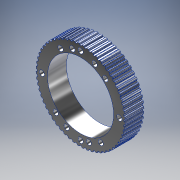
# Autodesk Inventor part: Synchronous Pulley1
Saved by Autodesk Inventor 2019.4 (Build 234330000, 330)
## iProperties
Created: 2019-11-30
Part Number: Synchronous Pulley1
Material: Aluminum 6061
Document SubType Name: Modeling
Designer: admin
Density: 2.7 g/cm^3
Appearance: Aluminum - Flat
Mass: 156.055 g
Surface Area: 190.164 cm^2
Volume: 57.7982 cm^3
CustomPartVersion: 1
Author: admin
Autodesk Inventor part; units mm, degrees
ref_plane "YZ Plane" through (0, 0, 0) normal (1, 0, 0) x (0, 1, 0)
ref_plane "XZ Plane" through (0, 0, 0) normal (0, 1, 0) x (-1, 0, 0)
ref_plane "XY Plane" through (0, 0, 0) normal (0, 0, 1) x (1, 0, 0)
sketch "Pulley Sketch" plane through (0, 0, 0) normal (0, 0, 1) x (1, 0, 0)
  circle A0 centre (0, 0) radius 47.7465 construction
  circle A1 centre (0, 0) radius 47.2465
  circle A2 centre (0, 0) radius 45.9965
  line L0 (-1.4722, 47.2235) -> (-0.9, 45.9965)
  line L1 (-0.9, 45.9965) -> (0.9, 45.9965)
  line L2 (0.9, 45.9965) -> (1.4722, 47.2235)
  line L3 (0, 0) -> (0, 47.2465) construction
  point P0 (0, 45.9965)
  dimension "d0" = 95.493
  dimension "d1" = 0.5
  dimension "d2" = 1.25
  dimension "d3" = 50
  dimension "d4" = 1.8
  constraints: 8 end point, 3 coincident, 3 point on circle, 2 centre point, 1 horizontal, 1 midpoint, 1 point on line, 1 vertical, 1 vertical alignment, 3 other
  measures "d0" diameter of A0
  measures "d1" radial gap between concentric circles of A0 A1
  measures "d3" angle of L2 L0
  measures "d4" distance of L0.end L1.end
extrude "Base Body" add sketch "Pulley Sketch" along normal mid plane 20 contours A2 | A1 L0 L1 L2 | L2 L1 L0 A1
extrude "Tooth" cut sketch "Pulley Sketch" along normal through all both and the other way through all contours L2 L1 L0 A1 picked at (0, 46.8281)
fillet "Tooth Fillet" radius 0.4 2 edges at (0.9, 45.9965, 0) (-0.9, 45.9965, 0)
fillet "Tooth Fillet" radius 0.6 4 edges at (-1.4722, 47.2235, 5) (-1.4722, 47.2235, -5) (1.4722, 47.2235, 5) (1.4722, 47.2235, -5)
pattern_circular "Teeth" count 60 over 360 about axis through (0, 0, -10) along (0, 0, 1) of "Tooth", "Tooth Fillet"
feature "Left flange" [suppressed]
feature "Right flange" [suppressed]
sketch "Sketch2" plane through (0, 0, 10) normal (0, 0, 1) x (1, 0, 0)
  arc A0 (-41.8204, 21.9837) -> (-42.3666, 20.9118) centre (0, 0) ccw projected
  constraints: 1 coincident
hole "Hole1" at (0, 0, 10) direction (0, 0, -1) diameter 70 end through all
sketch "Sketch3" plane through (0, 0, 10) normal (0, 0, 1) x (1, 0, 0)
  circle A0 centre (0, 41) radius 2.75
  line L0 (0, 41) -> (0, 0) construction
  circle A1 centre (-41, 0) radius 2.75
  circle A2 centre (0, -41) radius 2.75
  circle A3 centre (41, 0) radius 2.75
  dimension "d24" = 5.5
  dimension "d25" = 41
  dimension "d28" = 360
  constraints: 4 centre point, 2 end point, 1 vertical, 9 other
  measures "d24" diameter of A0
  measures "d25" distance of L0.start L0.end
extrude "Extrusion3" cut sketch "Sketch3" against normal through all
sketch "Sketch4" plane through (0, 0, -10) normal (0, 0, -1) x (-1, 0, 0)
  circle A0 centre (26.304, -28.5706) radius 2.75 projected
  circle A1 centre (14.887, -36.485) radius 2.75 projected
  circle A2 centre (-8.6878, -38.4357) radius 2.75 projected
  circle A3 centre (-21.2503, -32.5055) radius 2.75 projected
  circle A4 centre (21.2503, 32.5055) radius 2.75 projected
  circle A5 centre (8.6878, 38.4357) radius 2.75 projected
  circle A6 centre (-14.887, 36.485) radius 2.75 projected
  circle A7 centre (-26.304, 28.5706) radius 2.75 projected
  point P0 (0, 0)
extrude "Extrusion4" cut sketch "Sketch4" against normal through all
equation "\"d1\" = da_a"
equation "\"d2\" = da_hg"
equation "\"d3\" = 2 * da_fi"
equation "\"d4\" = da_bw"
equation "\"d5\" = da_bf"
equation "\"d7\" = da_bf"
equation "\"d9\" = da_rb"
equation "\"d10\" = da_rt"
equation "\"da_pb\" = 5"
equation "\"da_fi\" = 25deg"
equation "\"da_hg\" = 1.25"
equation "\"da_bw\" = 1.8"
equation "\"da_rb\" = 0.4"
equation "\"da_rt\" = 0.6"
equation "\"da_a\" = 0.5"
equation "\"da_bf\" = 20"
equation "\"da_wf\" = 2"
equation "\"da_hf\" = 3"
body "Solid1"
